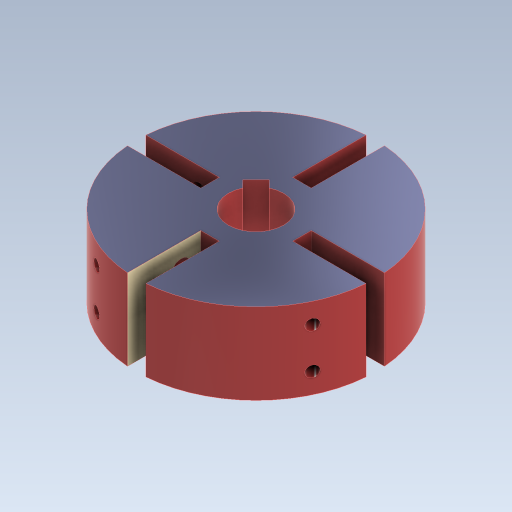
# Autodesk Inventor part: Pump-Motor-CW-Rotation:Rotor
Saved by Autodesk Inventor 2024.2 (Build 282272000, 272)
## iProperties
Created: 2025-06-16
Material: Aluminum 6061
Document SubType Name: Modeling
Density: 2.7 g/cm^3
Appearance: Red
Mass: 59.911 g
Surface Area: 155.769 cm^2
Volume: 59.911 cm^3
Designer: cw
Author: cw
Autodesk Inventor part; units mm, degrees
ref_plane "YZ Plane" through (0, 0, 0) normal (1, 0, 0) x (0, 1, 0)
sketch "Sketch1" plane through (0, 0, 0) normal (0, 0, 1) x (1, 0, 0)
  circle A0 centre (0, 0) radius 32.5
  dimension "d0" = 65
  constraints: 1 centre point, 1 coincident
  measures "d0" diameter of A0
extrude "Extrusion1" add sketch "Sketch1" along normal mid plane 22
sketch "Sketch2" plane through (0, 0, 11) normal (0, 0, 1) x (1, 0, 0)
  point P0 (0, 0)
hole "Hole1" at (0, 0, 11) direction (0, 0, -1) diameter 15 end through all
sketch "Sketch3" plane through (0, 0, 11) normal (0, 0, 1) x (1, 0, 0)
  circle A0 centre (0, 0) radius 32.5 projected
  line L0 (-32.4037, 2.5) -> (-12.5, 2.5)
  line L1 (-12.5, 2.5) -> (-12.5, -2.5)
  line L2 (-12.5, -2.5) -> (-32.4037, -2.5)
  point P0 (-12.5, 0)
  dimension "d10" = 5
  dimension "d11" = 12.5
  constraints: 6 end point, 2 perpendicular, 2 point on circle, 1 horizontal, 1 horizontal alignment, 1 midpoint
  measures "d10" distance between parallel lines of L2 L0
  measures "d11" distance from line of point (0, 0) L1
extrude "Extrusion2" cut sketch "Sketch3" against normal through all contours L0 L1 L2 A0 picked at (-19.1631, -0.278)
pattern_circular "Circular Pattern1" count 4 over 360 about axis through (0, 0, 0) along (0, 0, 1) of "Extrusion2"
ref_plane "Work Plane1" through (0, 0, 5.5) normal (0, 0, 1) x (1, 0, 0)
sketch "Sketch4" plane through (0, 0, 5.5) normal (0, 0, 1) x (1, 0, 0)
  line L0 (0, -45.3652) -> (0, 45.3652) construction
  arc A0 (32.4037, 2.5) -> (2.5, 32.4037) centre (0, 0) ccw projected
  line L1 (15.4072, 28.6159) -> (0, 13.2087)
  line L2 (0, 13.2087) -> (-1.0607, 14.2694)
  line L3 (-1.0607, 14.2694) -> (14.3465, 29.6765)
  line L4 (14.3465, 29.6765) -> (15.4072, 28.6159)
  point P0 (14, 29.33)
  dimension "d18" = 14
  dimension "d19" = 45
  dimension "d20" = 3
  constraints: 8 end point, 2 parallel, 2 point on circle, 2 point on line, 1 perpendicular
  measures "d18" distance from line of point (14, 29.33) L0
  measures "d19" angle of L3 L0
  measures "d20" diameter of L1 L3
revolve "Revolution1" cut sketch "Sketch4" angle 360 about axis through (-1.0607, 14.2694, 5.5) along (0.7071068, 0.7071068, 0)
pattern_linear "Rectangular Pattern1" count 2 spacing 11 along (0, 0, -1) of "Revolution1"
pattern_circular "Circular Pattern2" count 4 over 360 about axis through (0, 0, -10) along (0, 0, 1) of "Revolution1", "Rectangular Pattern1"
sketch "Sketch5" plane through (0, 0, 11) normal (0, 0, 1) x (1, 0, 0)
  line L0 (-45.3652, 0) -> (45.3652, 0) construction
  circle A0 centre (0, 0) radius 7.5 projected
  line L1 (-3.2322, 6.7678) -> (-5.1619, 8.6974)
  line L2 (-5.1619, 8.6974) -> (-8.6974, 5.1619)
  line L3 (-8.6974, 5.1619) -> (-6.7678, 3.2322)
  line L4 (0, 0) -> (-6.9296, 6.9296) construction
  dimension "d28" = 45
  dimension "d29" = 5
  dimension "d31" = 17.3
  constraints: 8 end point, 2 parallel, 2 point on circle, 1 midpoint, 1 perpendicular
  measures "d28" angle of L0 L4
  measures "d29" distance between parallel lines of L1 L3
extrude "Extrusion3" cut sketch "Sketch5" against normal through all contours A0 L3 L2 L1
ref_plane "Work Plane2" through (-6.9296, 6.9296, -11) normal (0.7071068, 0.7071068, 0) x (-0.7071068, 0.7071068, 0)
body "Solid1"
